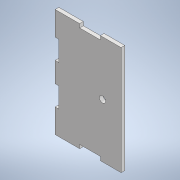
# Autodesk Inventor part: top switch
Saved by Autodesk Inventor 2020 (Build 240168000, 168)
## iProperties
Created: 2022-02-16
Part Number: top switch
Material: Generic
Document SubType Name: Modeling
Designer: rwte
Density: 1 g/cm^3
Appearance: Default
Author: rwte
Autodesk Inventor part; units mm, degrees
ref_plane "YZ Plane" through (0, 0, 0) normal (1, 0, 0) x (0, 1, 0)
ref_plane "XZ Plane" through (0, 0, 0) normal (0, 1, 0) x (-1, 0, 0)
ref_plane "XY Plane" through (0, 0, 0) normal (0, 0, 1) x (1, 0, 0)
sketch "Sketch1" plane through (0, 0, 0) normal (0, 0, 1) x (1, 0, 0)
  line L0 (-25, -40.5) -> (-25, 40.5)
  line L1 (-25, 40.5) -> (25, 40.5)
  line L2 (25, 40.5) -> (25, -40.5)
  line L3 (25, -40.5) -> (-25, -40.5)
  line L4 (-25, -40.5) -> (25, 40.5) construction
  line L5 (-25, 40.5) -> (25, -40.5) construction
  line L6 (-25, 40.5) -> (-8.3333, 40.5)
  line L7 (-8.3333, 40.5) -> (-8.3333, 43.5)
  line L8 (-8.3333, 43.5) -> (-25, 43.5)
  line L9 (-25, 43.5) -> (-25, 40.5) construction
  line L10 (25, 40.5) -> (8.3333, 40.5)
  line L11 (8.3333, 40.5) -> (8.3333, 43.5)
  line L12 (8.3333, 43.5) -> (25, 43.5)
  line L13 (25, 43.5) -> (25, 40.5)
  line L14 (-38.6, 0) -> (35.6, 0) projected
  line L15 (0, -60.9) -> (0, 60.9) projected
  line L16 (-8.3333, -40.5) -> (-8.3333, -43.5)
  line L17 (-8.3333, -43.5) -> (-25, -43.5)
  line L18 (-25, -43.5) -> (-25, -40.5) construction
  line L19 (8.3333, -40.5) -> (8.3333, -43.5)
  line L20 (8.3333, -43.5) -> (25, -43.5)
  line L21 (25, -43.5) -> (25, -40.5)
  line L22 (-25, -40.5) -> (-25, -24.3)
  line L23 (-25, -24.3) -> (-28, -24.3)
  line L24 (-28, -24.3) -> (-28, -40.5)
  line L25 (-28, -40.5) -> (-25, -40.5) construction
  line L26 (-25, -8.1) -> (-25, 8.1)
  line L27 (-25, 8.1) -> (-28, 8.1)
  line L28 (-28, 8.1) -> (-28, -8.1)
  line L29 (-28, -8.1) -> (-25, -8.1)
  line L30 (-25, 40.5) -> (-25, 24.3)
  line L31 (-25, 24.3) -> (-28, 24.3)
  line L32 (-28, 24.3) -> (-28, 40.5)
  line L33 (-28, 40.5) -> (-25, 40.5) construction
  line L34 (-25, 43.5) -> (-28, 43.5)
  line L35 (-28, 43.5) -> (-28, 40.5)
  line L36 (-25, -43.5) -> (-28, -43.5)
  line L37 (-28, -43.5) -> (-28, -40.5)
  point P0 (0, 0)
  point P1 (16.6667, 43.5)
  point P2 (-16.6667, 43.5)
  point P3 (16.6667, -43.5)
  point P4 (-16.6667, -43.5)
  point P5 (-28, 32.4)
  point P6 (-28, 0)
  point P7 (-28, -32.4)
  point P8 (-25, 0)
  dimension "d0" = 81
  dimension "d1" = 50
  dimension "d4" = 16.6667
  dimension "d5" = 16.6667
  dimension "d6" = 3
  dimension "d7" = 3
  dimension "d8" = 16.2
  constraints: 72 end point, 12 parallel, 9 perpendicular, 8 midpoint, 8 symmetric about line, 7 point on line, 2 collinear, 2 horizontal alignment, 2 vertical alignment, 1 horizontal, 1 vertical
  measures "d0" distance of L1.end L2.end
  measures "d1" distance of L0.end L1.end
  measures "d4" distance of L8.end L7.end
  measures "d5" distance of L12.end L11.end
  measures "d6" distance of L1.end L12.end
  measures "d7" distance of L32.end L0.end
  measures "d8" distance of L31.end L32.end
extrude "Extrusion1" add sketch "Sketch1" along normal blind 3
sketch "Sketch2" plane through (0, 0, 3) normal (0, 0, 1) x (1, 0, 0)
  line L0 (-38.6, 0) -> (35.6, 0) projected
  line L1 (0, -60.9) -> (0, 60.9) projected
  circle A0 centre (10, 0) radius 2.5
  line L2 (25, -43.5) -> (25, 43.5) projected
  dimension "d9" = 5
  dimension "d12" = 15
  constraints: 1 centre point, 1 coincident, 1 point on line, 1 other
  measures "d9" diameter of A0
  measures "d12" distance from line of L2 point (10, 0)
extrude "Extrusion2" cut sketch "Sketch2" against normal through all
equation "\"d4\" = 0.333333 * d1"
equation "\"d5\" = d4"
equation "\"d6\" = d2"
equation "\"d7\" = d2"
equation "\"d8\" = 0.2 * d0"
equation "\"d2\" = 3"
body "Solid1"
